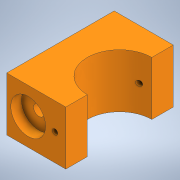
# Autodesk Inventor part: acople_tubo
Saved by Autodesk Inventor 2022 (Build 260153000, 153)
## iProperties
Created: 2022-01-28
Part Number: acople_tubo
Material: Generic
Document SubType Name: Modeling
Designer: Home
Density: 1 g/cm^3
Appearance: Default
Author: Home
Autodesk Inventor part; units mm, degrees
ref_plane "YZ Plane" through (0, 0, 0) normal (1, 0, 0) x (0, 1, 0)
ref_plane "XZ Plane" through (0, 0, 0) normal (0, 1, 0) x (-1, 0, 0)
ref_plane "XY Plane" through (0, 0, 0) normal (0, 0, 1) x (1, 0, 0)
sketch "Sketch1" plane through (0, 0, 0) normal (0, 1, 0) x (-1, 0, 0)
  line L0 (0, -50) -> (55, -50)
  line L1 (55, -50) -> (55, 50)
  line L2 (55, 50) -> (0, 50)
  arc A0 (0, -30) -> (0, 30) centre (0, 0) ccw
  line L3 (0, 50) -> (0, 30)
  line L4 (0, -30) -> (0, -50)
  point P0 (55, 0)
  dimension "d0" = 100
  dimension "d1" = 55
  dimension "d3" = 60
  constraints: 10 end point, 3 parallel, 2 coincident, 2 point on circle, 2 vertical alignment, 1 centre point, 1 horizontal, 1 horizontal alignment, 1 midpoint, 1 perpendicular
  measures "d0" distance of L0.end L1.end
  measures "d1" distance of L1.end L2.end
  measures "d3" diameter of A0
extrude "Extrusion1" add sketch "Sketch1" along normal blind 50
sketch "Sketch2" plane through (-55, 0, 50) normal (0, 0, 1) x (1, 0, 0)
  line L0 (55, 0) -> (55, 50) construction
  line L1 (55, 50) -> (0, 50) construction
  line L2 (55, 0) -> (0, 0) construction
  line L3 (0, 0) -> (0, 50) projected
  point P0 (20, 25)
  point P1 (0, 25)
  dimension "d14" = 20
  constraints: 1 horizontal alignment, 1 midpoint
  measures "d14" distance from line of L3 point (20, 25)
hole "Hole1" at (-35, 25, 50) direction (0, 0, -1) diameter 10 end through all counterbore diameter 32.4 counterbore depth 10
sketch "Sketch4" plane through (0, 0, -50) normal (0, 0, -1) x (-1, 0, 0)
  line L0 (55, 0) -> (55, 50) projected
  line L1 (0, 0) -> (0, 50) projected
  point P0 (10, 25)
  point P1 (55, 25)
  dimension "d15" = 10
  constraints: 1 horizontal alignment, 1 midpoint
  measures "d15" distance from line of L1 point (10, 25)
hole "Hole2" at (-10, 25, -50) direction (0, 0, 1) diameter 5 end through all
body "Solid1"
